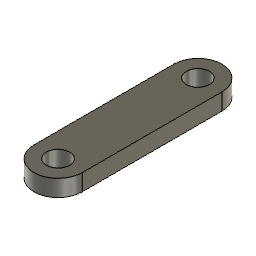
Slider to Claw arm (Autodesk Fusion 360 design; units mm, degrees)
Autodesk Fusion 360 part; units mm, degrees
sketch "Sketch1" plane through (0, 0, 0) normal (0, 0, 1) x (1, 0, 0)
  line L0 (0, 0) -> (0, 33.32) construction
  line L1 (0, 33.32) -> (0, 33.325) construction
  circle A0 centre (0, 33.325) radius 2.75
  circle A1 centre (0, 0) radius 2.75
  circle A2 centre (0, 0) radius 5.75
  circle A3 centre (0, 33.325) radius 5.75
  line L2 (0, 33.325) -> (-5.75, 33.325) construction
  line L3 (0, 33.325) -> (5.75, 33.325) construction
  line L4 (0, 0) -> (5.75, 0) construction
  line L5 (0, 0) -> (-5.75, 0) construction
  line L6 (-5.75, 0) -> (-5.75, 33.325)
  line L7 (5.75, 0) -> (5.75, 33.325)
  dimension "d1" = 33.32
  dimension "d2" = 0.005
  dimension "d3" = 5.5
  dimension "d4" = 5.5
  dimension "d5" = 11.5
  dimension "d6" = 11.5
  constraint coincident L0.start A1.centre
  constraint vertical L0
  constraint vertical L1
  constraint coincident L1.end A0.centre
  constraint concentric A1 A2
  constraint concentric A0 A3
  constraint coincident A3 L2.end
  constraint perpendicular L0 L2
  constraint coincident A3 L3.end
  constraint parallel L2 L3
  constraint coincident A2 L4.end
  constraint perpendicular L0 L4
  constraint coincident A2 L5.end
  constraint perpendicular L0 L5
  measures "d1" distance of L0.start L0.end
  measures "d2" distance of L0.end L1.end
  measures "d3" diameter of A0
  measures "d4" diameter of A1
  measures "d5" diameter of A2
  measures "d6" diameter of A3
extrude "Extrude1" add sketch "Sketch1" along normal blind 4
